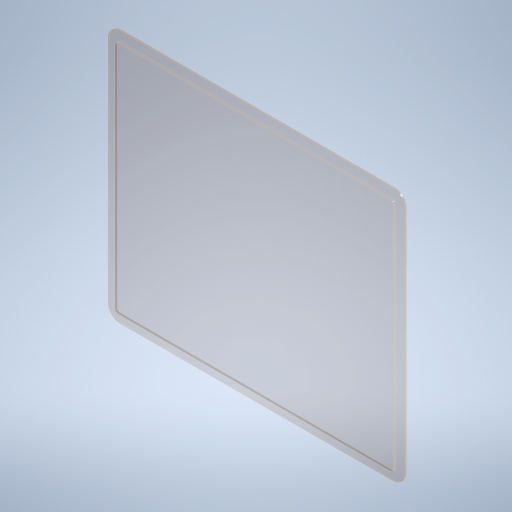
# Autodesk Inventor part: Door Window
Saved by Autodesk Inventor 2024 (Build 280153000, 153)
## iProperties
Created: 2024-12-01
Part Number: Door Window
Material: Polycarbonate, Smoke
Document SubType Name: Modeling
Designer: Ishaan
Density: 1.2 g/cm^3
Appearance: Polycarbonate - Smoked
Author: Ishaan
Autodesk Inventor part; units mm, degrees
ref_plane "YZ Plane" through (0, 0, 0) normal (1, 0, 0) x (0, 1, 0)
ref_plane "XZ Plane" through (0, 0, 0) normal (0, 1, 0) x (-1, 0, 0)
sketch "Sketch1" plane through (0, 0, 0) normal (0, 0, 1) x (1, 0, 0)
  line L0 (176.5, -149) -> (-176.5, -149)
  line L1 (-176.5, -149) -> (-176.5, 149)
  line L2 (-176.5, 149) -> (176.5, 149)
  line L3 (176.5, 149) -> (176.5, -149)
  line L4 (176.5, -149) -> (-176.5, 149) construction
  line L5 (-176.5, -149) -> (176.5, 149) construction
  point P0 (0, 0)
  dimension "d0" = 353
  dimension "d1" = 298
  constraints: 12 end point, 2 midpoint, 2 parallel, 1 horizontal, 1 perpendicular
  measures "d0" distance of L1.end L2.end
  measures "d1" distance of L0.end L1.end
extrude "Extrusion1" add sketch "Sketch1" along normal blind 4.7625
fillet "Fillet1" radius 4 4 edges at (-176.5, -149, 2.3813) (176.5, -149, 2.3813) (176.5, 149, 2.3813) (-176.5, 149, 2.3813)
sketch "Sketch2" plane through (0, 0, 4.7625) normal (0, 0, 1) x (1, 0, 0)
  arc A0 (-172.5, 149) -> (-176.5, 145) centre (-172.5, 145) ccw projected
  line L0 (-176.5, 145) -> (-176.5, -145) projected
  arc A1 (-176.5, -145) -> (-172.5, -149) centre (-172.5, -145) ccw projected
  line L1 (-172.5, -149) -> (172.5, -149) projected
  arc A2 (172.5, -149) -> (176.5, -145) centre (172.5, -145) ccw projected
  line L2 (176.5, -145) -> (176.5, 145) projected
  arc A3 (176.5, 145) -> (172.5, 149) centre (172.5, 145) ccw projected
  line L3 (172.5, 149) -> (-172.5, 149) projected
  arc A4 (-172.5, 148.5) -> (-176, 145) centre (-172.5, 145) ccw
  line L4 (-176, 145) -> (-176, -145)
  arc A5 (-176, -145) -> (-172.5, -148.5) centre (-172.5, -145) ccw
  line L5 (-172.5, -148.5) -> (172.5, -148.5)
  arc A6 (172.5, -148.5) -> (176, -145) centre (172.5, -145) ccw
  line L6 (176, -145) -> (176, 145)
  arc A7 (176, 145) -> (172.5, 148.5) centre (172.5, 145) ccw
  line L7 (172.5, 148.5) -> (-172.5, 148.5)
  point P0 (0, 0)
  dimension "d5" = 0.5
  constraints: 8 end point, 8 point on circle, 4 centre point, 7 other
  measures "d5" distance between parallel lines of L3 L7
extrude "Extrusion2" cut sketch "Sketch2" against normal through all
sketch "Sketch3" plane through (0, 0, 0) normal (0, 0, -1) x (-1, 0, 0)
  arc A0 (-172.5, 148.5) -> (-176, 145) centre (-172.5, 145) ccw projected
  line L0 (-176, 145) -> (-176, -145) projected
  arc A1 (-176, -145) -> (-172.5, -148.5) centre (-172.5, -145) ccw projected
  line L1 (-172.5, -148.5) -> (172.5, -148.5) projected
  arc A2 (172.5, -148.5) -> (176, -145) centre (172.5, -145) ccw projected
  line L2 (176, -145) -> (176, 145) projected
  arc A3 (176, 145) -> (172.5, 148.5) centre (172.5, 145) ccw projected
  line L3 (172.5, 148.5) -> (-172.5, 148.5) projected
  arc A4 (-172.5, 160.5) -> (-188, 145) centre (-172.5, 145) ccw
  line L4 (-188, 145) -> (-188, -145)
  arc A5 (-188, -145) -> (-172.5, -160.5) centre (-172.5, -145) ccw
  line L5 (-172.5, -160.5) -> (172.5, -160.5)
  arc A6 (172.5, -160.5) -> (188, -145) centre (172.5, -145) ccw
  line L6 (188, -145) -> (188, 145)
  arc A7 (188, 145) -> (172.5, 160.5) centre (172.5, 145) ccw
  line L7 (172.5, 160.5) -> (-172.5, 160.5)
  point P0 (0, 0)
  dimension "d8" = 12
  constraints: 8 end point, 8 point on circle, 4 centre point, 7 other
  measures "d8" distance between parallel lines of L3 L7
ref_plane "Work Plane1" through (0, 0, 1.7625) normal (0, 0, 1) x (1, 0, 0)
extrude "Extrusion3" add sketch "Sketch3" against normal up to surface (1.7625 mm away)
body "Solid1"
